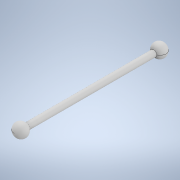
# Autodesk Inventor part: PX9200-28
Saved by Autodesk Inventor 2022.3 (Build 263350000, 350)
## iProperties
Created: 2022-07-15
Part Number: PX9200-28
Material: Generic
Document SubType Name: Modeling
Designer: luis_
Density: 1 g/cm^3
Appearance: Default
Author: luis_
Autodesk Inventor part; units mm, degrees
ref_plane "YZ Plane" through (0, 0, 0) normal (1, 0, 0) x (0, 1, 0)
ref_plane "XZ Plane" through (0, 0, 0) normal (0, 1, 0) x (-1, 0, 0)
ref_plane "XY Plane" through (0, 0, 0) normal (0, 0, 1) x (1, 0, 0)
sketch "Sketch2" plane through (0, 0, 0) normal (0, 0, 1) x (1, 0, 0)
  circle A0 centre (0, 0) radius 1.5
  dimension "d6" = 3
  constraints: 1 centre point, 1 coincident
  measures "d6" diameter of A0
extrude "Extrusion1" add sketch "Sketch2" along normal blind 61
sketch "Sketch3" plane through (0, 0, 0) normal (0, 1, 0) x (-1, 0, 0)
  line L0 (1.5, 61) -> (-1.5, 61) projected
  ellipse E0 centre (0, 63.71) end of major axis (0, 60.71) minor radius 3.2451
  ellipse E1 centre (0, -2.714) end of major axis (0, -5.714) minor radius 3.2451
  line L1 (0, 61) -> (0, 66.71)
  line L2 (0, -5.714) -> (0, 0)
  line L3 (1.5, 0) -> (-1.5, 0) projected
  point P0 (1.392, 61)
  point P1 (-1.3828, 0)
  dimension "d11" = 2.71
  constraints: 4 end point, 2 coincident, 2 midpoint, 1 vertical, 6 other
  measures "d11" distance from line of L0 point (0, 63.71)
revolve "Revolution1" add sketch "Sketch3" angle 360 about axis through (0, 0, 61) along (0, 0, 1) picked at (0.8466, 64.635) contours L0 L1 E0
revolve "Revolution2" add sketch "Sketch3" angle 360 about axis through (0, 0, -5.714) along (0, 0, 1) picked at (-0.7775, -3.6647) contours E1 L3 L2
body "Solid1"
